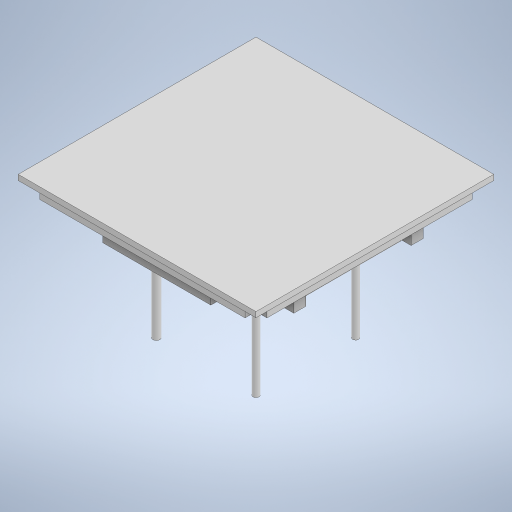
# Autodesk Inventor part: Acrilico_Bottom
Saved by Autodesk Inventor 2024 (Build 280153000, 153)
## iProperties
Created: 2023-06-25
Part Number: Acrilico_Bottom
Material: Genérico
Document SubType Name: Modeling
Designer: Personal
Density: 2.56911 g/cm^3
Appearance: Valor por defecto
Mass: 906.6 g
Surface Area: 1709.61 cm^2
Volume: 352.885 cm^3
Author: Personal
Autodesk Inventor part; units mm, degrees
ref_plane "YZ Plane" through (0, 0, 0) normal (1, 0, 0) x (0, 1, 0)
ref_plane "XZ Plane" through (0, 0, 0) normal (0, 1, 0) x (-1, 0, 0)
ref_plane "XY Plane" through (0, 0, 0) normal (0, 0, 1) x (1, 0, 0)
sketch "Boceto1" plane through (0, 0, 0) normal (0, 1, 0) x (-1, 0, 0)
  line L0 (-97.5, 97.5) -> (97.5, 97.5)
  line L1 (97.5, 97.5) -> (97.5, -97.5)
  line L2 (97.5, -97.5) -> (-97.5, -97.5)
  line L3 (-97.5, -97.5) -> (-97.5, 97.5)
  line L4 (-97.5, 97.5) -> (97.5, -97.5) construction
  line L5 (97.5, 97.5) -> (-97.5, -97.5) construction
  point P0 (0, 0)
  dimension "d0" = 195
  dimension "d1" = 195
  constraints: 12 end point, 2 midpoint, 2 parallel, 1 horizontal, 1 perpendicular
  measures "d0" distance of L0.end L1.end
  measures "d1" distance of L0.start L0.end
extrude "Extrusión1" add sketch "Boceto1" along normal mid plane 4.4
sketch "Boceto4" plane through (0, -2.2, 0) normal (0, -1, 0) x (1, 0, 0)
  line L0 (97.5, -97.5) -> (97.5, 97.5) construction
  line L1 (-97.5, 97.5) -> (-97.5, -97.5) construction
  line L2 (84.1, -93.1) -> (-84.1, -93.1)
  line L3 (-84.1, -93.1) -> (-84.1, -84.1)
  line L4 (-84.1, -84.1) -> (84.1, -84.1)
  line L5 (84.1, -84.1) -> (84.1, -93.1)
  line L6 (-97.5, -97.5) -> (97.5, -97.5) construction
  line L7 (93.1, -84.1) -> (84.1, -84.1)
  line L8 (84.1, -84.1) -> (84.1, 84.1)
  line L9 (84.1, 84.1) -> (93.1, 84.1)
  line L10 (93.1, 84.1) -> (93.1, -84.1)
  line L11 (0, -126.8945) -> (0, 107.949)
  line L12 (-84.1, -84.1) -> (-84.1, 84.1)
  line L13 (-84.1, 84.1) -> (-93.1, 84.1)
  line L14 (-93.1, 84.1) -> (-93.1, -84.1)
  line L15 (-93.1, -84.1) -> (-84.1, -84.1)
  line L16 (84.1, 84.1) -> (-84.1, 84.1)
  line L17 (84.1, 93.1) -> (-84.1, 93.1)
  line L18 (84.1, 84.1) -> (84.1, 93.1)
  line L19 (-84.1, 84.1) -> (-84.1, 93.1)
  point P0 (0, 0)
  point P1 (-84.1, -88.6)
  point P2 (88.6, -84.1)
  point P3 (84.1, -84.1)
  point P4 (84.1, -84.1)
  point P5 (84.1, -84.1)
  point P6 (84.1, -84.1)
  point P7 (-84.1, 84.1)
  point P8 (-84.1, 84.1)
  point P9 (-84.1, 84.1)
  point P10 (-84.1, 84.1)
  dimension "d20" = 4.4
  dimension "d21" = 9
  dimension "d22" = 13.4
  dimension "d23" = 13.4
  dimension "d24" = 4.4
  dimension "d25" = 9
  dimension "d26" = 13.4
  dimension "d30" = 9
  constraints: 34 end point, 5 horizontal, 4 parallel, 4 symmetric about line, 3 vertical, 2 midpoint, 2 perpendicular
  measures "d20" distance between parallel lines of L2 L6
  measures "d21" distance of L4.end L2.start
  measures "d22" distance between parallel lines of L0 L5
  measures "d23" distance from line of L1 point (-84.1, -88.6)
  measures "d24" distance between parallel lines of L0 L10
  measures "d25" distance of L7.start L7.end
  measures "d26" distance from line of point (88.6, -84.1) L6
  measures "d30" distance between parallel lines of L17 L16
extrude "Extrusión6" add sketch "Boceto4" along normal blind 9 contours L2 L11 L4 L5 | L2 L3 L4 L11 | L8 L9 L10 L7 | L16 L11 L17 L18 | L15 L14 L13 L12 | L16 L19 L17 L11
sketch "Boceto5" plane through (0, -11.2, 0) normal (0, -1, 0) x (1, 0, 0)
  line L0 (-84.1, -93.1) -> (84.1, -93.1) construction
  line L1 (93.1, -84.1) -> (93.1, 84.1) construction
  line L2 (-93.1, 84.1) -> (-93.1, -84.1) construction
  line L3 (84.1, 93.1) -> (-84.1, 93.1) construction
  line L4 (84.1, -93.1) -> (-84.1, -93.1)
  line L5 (-93.1, -84.1) -> (-93.1, 84.1)
  line L6 (-84.1, 93.1) -> (84.1, 93.1)
  line L7 (93.1, 84.1) -> (93.1, -84.1)
  line L8 (84.1, -93.1) -> (84.1, -84.1) projected
  line L9 (84.1, -84.1) -> (-84.1, -84.1) construction
  line L10 (84.1, -93.1) -> (84.1, -84.1)
  line L11 (84.1, -84.1) -> (93.1, -84.1)
  line L12 (93.1, 84.1) -> (84.1, 84.1)
  line L13 (84.1, 84.1) -> (84.1, 93.1)
  line L14 (-93.1, 84.1) -> (-84.1, 84.1)
  line L15 (-84.1, 84.1) -> (-84.1, 93.1)
  line L16 (-93.1, -84.1) -> (-84.1, -84.1) projected
  line L17 (-84.1, -93.1) -> (-84.1, -84.1)
  line L18 (-84.1, -84.1) -> (-93.1, -84.1)
  point P0 (0, 0)
  constraints: 24 end point, 9 point on line, 5 perpendicular, 2 horizontal, 2 parallel, 2 vertical
extrude "Extrusión7" add sketch "Boceto5" along normal blind 1.65
sketch "Boceto6" plane through (0, -12.85, 0) normal (0, -1, 0) x (1, 0, 0)
  line L0 (-84.1, -84.1) -> (84.1, -84.1) construction
  line L1 (53.1, -84.1) -> (43.1, -84.1)
  line L2 (43.1, -84.1) -> (43.1, -64.1)
  line L3 (43.1, -64.1) -> (53.1, -64.1)
  line L4 (53.1, -64.1) -> (53.1, -84.1)
  line L5 (93.1, -84.1) -> (93.1, 84.1) projected
  line L6 (84.1, -84.1) -> (84.1, 84.1) projected
  line L7 (64.1, -53.1) -> (84.1, -53.1)
  line L8 (84.1, -53.1) -> (84.1, -43.1)
  line L9 (84.1, -43.1) -> (64.1, -43.1)
  line L10 (64.1, -43.1) -> (64.1, -53.1)
  line L11 (-84.1, -93.1) -> (84.1, -93.1) projected
  point P0 (0, 0)
  dimension "d35" = 40
  dimension "d36" = 10
  dimension "d37" = 20
  dimension "d38" = 40
  dimension "d39" = 10
  dimension "d40" = 20
  constraints: 16 end point, 4 parallel, 2 horizontal, 2 perpendicular, 2 point on line
  measures "d35" distance between parallel lines of L5 L4
  measures "d36" distance of L2.end L3.end
  measures "d37" distance of L3.end L1.start
  measures "d38" distance between parallel lines of L11 L7
  measures "d39" distance of L9.end L7.start
  measures "d40" distance of L7.start L7.end
extrude "Extrusión8" add sketch "Boceto6" along normal blind 15
sketch "Boceto7" plane through (43.1, -12.85, -84.1) normal (-1, 0, 0) x (0, 0, 1)
  line L0 (0, 0) -> (20, 0) projected
  line L1 (0, 0) -> (0, -15) construction
  line L2 (20, -15) -> (0, -15) construction
  line L3 (20, 0) -> (20, -15) construction
  line L4 (0, 0) -> (20, 0) projected
  circle A0 centre (10, -7.5) radius 3.85
  point P0 (84.1, 12.85)
  dimension "d43" = 7.7
  constraints: 1 centre point
  measures "d43" diameter of A0
extrude "Extrusión9" add sketch "Boceto7" along normal blind 4
sketch "Boceto8" plane through (39.1, -20.35, -74.1) normal (-1, 0, 0) x (0, 0, 1)
  circle A0 centre (0, 0) radius 3.85 projected
  circle A1 centre (0, 0) radius 7.25
  point P0 (74.1, 20.35)
  dimension "d46" = 14.5
  constraints: 1 centre point, 1 coincident
  measures "d46" diameter of A1
extrude "Extrusión10" add sketch "Boceto8" along normal up to surface (39.1 mm away)
sketch "Boceto10" plane through (39.1, -20.35, -74.1) normal (-1, 0, 0) x (0, 0, 1)
  circle A0 centre (0, 0) radius 3.85 projected
  point P0 (74.1, 20.35)
extrude "Extrusión11" add sketch "Boceto10" along normal up to surface (39.1 mm away)
mirror "Simetría4" about plane through (0, 0, 0) normal (1, 0, 0) of "Extrusión9", "Extrusión10", "Extrusión11", "Extrusión8"
sketch "Boceto11" plane through (-84.1, -27.85, -53.1) normal (0, -1, 0) x (1, 0, 0)
  line L0 (20, 0) -> (0, 0) projected
  line L1 (20, 10) -> (20, 0) projected
  line L2 (0, 10) -> (20, 10) projected
  line L3 (0, 0) -> (0, 10) projected
  point P0 (84.1, 53.1)
extrude "Extrusión12" cut sketch "Boceto11" against normal up to surface (15 mm away)
sketch "Boceto12" plane through (64.1, -12.85, -43.1) normal (0, 0, 1) x (1, 0, 0)
  line L0 (0, 0) -> (20, 0) projected
  line L1 (0, 0) -> (0, -15) projected
  line L2 (20, -15) -> (0, -15) projected
  line L3 (20, 0) -> (20, -15) projected
  circle A0 centre (10, -7.5) radius 3.85
  point P0 (-64.1, 12.85)
  dimension "d53" = 7.7
  constraints: 1 centre point
  measures "d53" diameter of A0
extrude "Extrusión13" add sketch "Boceto12" along normal blind 4 contours A0
sketch "Boceto13" plane through (74.1, -20.35, -39.1) normal (0, 0, 1) x (1, 0, 0)
  circle A0 centre (0, 0) radius 3.85 projected
  circle A1 centre (0, 0) radius 7.25
  point P0 (-74.1, 20.35)
  dimension "d56" = 14.5
  constraints: 1 centre point, 1 coincident
  measures "d56" diameter of A1
extrude "Extrusión14" add sketch "Boceto13" along normal up to surface (39.1 mm away)
sketch "Boceto14" plane through (74.1, -20.35, -39.1) normal (0, 0, 1) x (1, 0, 0)
  circle A0 centre (0, 0) radius 3.85 projected
  point P0 (-74.1, 20.35)
extrude "Extrusión15" add sketch "Boceto14" along normal up to surface (39.1 mm away)
mirror "Simetría5" about plane through (0, 0, 0) normal (0, 0, 1) of "Extrusión15", "Extrusión14", "Extrusión13", "Extrusión12", "Extrusión8"
sketch "Boceto15" plane through (43.1, -27.85, 64.1) normal (0, -1, 0) x (1, 0, 0)
  line L0 (10, 0) -> (0, 0) projected
  line L1 (10, 20) -> (10, 0) projected
  line L2 (0, 20) -> (10, 20) projected
  line L3 (0, 0) -> (0, 20) projected
  point P0 (-43.1, -64.1)
extrude "Extrusión16" cut sketch "Boceto15" against normal up to surface (15 mm away)
sketch "Boceto16" plane through (0, -12.85, 0) normal (0, -1, 0) x (1, 0, 0)
  line L0 (81.35, 39.1) -> (66.85, 39.1) construction
  line L1 (81.35, -39.1) -> (66.85, -39.1) construction
  line L2 (81.35, -39.1) -> (81.35, 39.1) construction
  line L3 (66.85, -39.1) -> (66.85, 39.1) construction
  line L4 (81.35, -39.1) -> (66.85, -39.1) construction
  line L5 (81.35, 39.1) -> (66.85, 39.1) construction
  line L6 (-39.1, -66.85) -> (-39.1, -81.35) projected
  line L7 (39.1, -66.85) -> (39.1, -81.35) projected
  line L8 (-81.35, -44.335) -> (-66.85, -44.335)
  line L9 (-66.85, -44.335) -> (-66.85, 44.335)
  line L10 (-66.85, 44.335) -> (-81.35, 44.335)
  line L11 (-81.35, 44.335) -> (-81.35, -44.335)
  line L12 (-93.1, 84.1) -> (-93.1, -84.1) construction
  line L13 (84.1, 93.1) -> (-84.1, 93.1) construction
  line L14 (-44.335, 81.35) -> (-44.335, 66.85)
  line L15 (-44.335, 66.85) -> (44.335, 66.85)
  line L16 (44.335, 66.85) -> (44.335, 81.35)
  line L17 (44.335, 81.35) -> (-44.335, 81.35)
  point P0 (0, 0)
  dimension "d84" = 11.75
  dimension "d85" = 14.5
  dimension "d86" = 88.67
  dimension "d87" = 48.765
  dimension "d88" = 14.5
  dimension "d89" = 88.67
  dimension "d90" = 48.765
  dimension "d91" = 11.75
  constraints: 20 end point, 4 coincident, 4 parallel, 2 perpendicular, 1 horizontal
  measures "d84" distance between parallel lines of L11 L12
  measures "d85" distance of L8.start L8.end
  measures "d86" distance of L8.end L9.end
  measures "d87" distance between parallel lines of L13 L10
  measures "d88" distance of L14.start L15.start
  measures "d89" distance of L15.start L15.end
  measures "d90" distance between parallel lines of L12 L14
  measures "d91" distance between parallel lines of L13 L17
sketch "Boceto17" plane through (0, -12.85, 0) normal (0, -1, 0) x (1, 0, 0)
  line L0 (50.85, 50.85) -> (-50.85, 50.85) construction
  line L1 (-50.85, 50.85) -> (-50.85, -50.85) construction
  line L2 (-50.85, -50.85) -> (50.85, -50.85) construction
  line L3 (50.85, -50.85) -> (50.85, 50.85) construction
  line L4 (50.85, 50.85) -> (-50.85, -50.85) construction
  line L5 (-50.85, 50.85) -> (50.85, -50.85) construction
  circle A0 centre (40.85, 40.85) radius 2.5
  circle A1 centre (-40.85, 40.85) radius 2.8882
  line L6 (101.7, 0) -> (-109.1959, 0)
  circle A2 centre (40.85, -40.85) radius 2.5
  circle A3 centre (-40.85, -40.85) radius 2.8882
  point P0 (0, 0)
  dimension "d67" = 101.7
  dimension "d68" = 101.7
  dimension "d69" = 5
  dimension "d70" = 10
  dimension "d71" = 10
  dimension "d72" = 10
  dimension "d73" = 10
  constraints: 14 end point, 4 centre point, 2 horizontal, 2 midpoint, 2 parallel, 2 symmetric about line, 1 perpendicular, 2 other
  measures "d67" distance of L1.end L2.end
  measures "d68" distance of L2.end L0.start
  measures "d69" diameter of A0
  measures "d70" distance from line of L3 A0.centre
  measures "d71" distance from line of L0 A0.centre
  measures "d72" distance from line of L0 A1.centre
  measures "d73" distance from line of L1 A1.centre
extrude "Extrusión19" add sketch "Boceto17" along normal blind 100.95
sketch "Boceto18" plane through (0, -12.85, 0) normal (0, -1, 0) x (1, 0, 0)
  line L0 (84.1, 93.1) -> (-84.1, 93.1) projected
  line L1 (-84.1, 93.1) -> (-84.1, 84.1) projected
  line L2 (-84.1, 84.1) -> (-93.1, 84.1) projected
  line L3 (-93.1, 84.1) -> (-93.1, -84.1) projected
  line L4 (-93.1, -84.1) -> (-84.1, -84.1) projected
  line L5 (-84.1, -84.1) -> (-84.1, -93.1) projected
  line L6 (-84.1, -93.1) -> (84.1, -93.1) projected
  line L7 (84.1, -93.1) -> (84.1, -84.1) projected
  line L8 (93.1, -84.1) -> (93.1, 84.1) projected
  line L9 (84.1, -84.1) -> (93.1, -84.1) projected
  line L10 (93.1, 84.1) -> (84.1, 84.1) projected
  line L11 (84.1, 84.1) -> (84.1, 93.1) projected
  line L12 (-81.0533, 90.0533) -> (81.0533, 90.0533)
  line L13 (81.0533, 90.0533) -> (81.0533, 81.0533)
  line L14 (81.0533, 81.0533) -> (90.0533, 81.0533)
  line L15 (90.0533, 81.0533) -> (90.0533, -81.0533)
  line L16 (90.0533, -81.0533) -> (81.0533, -81.0533)
  line L17 (81.0533, -81.0533) -> (81.0533, -90.0533)
  line L18 (81.0533, -90.0533) -> (-81.0533, -90.0533)
  line L19 (-81.0533, -90.0533) -> (-81.0533, -81.0533)
  line L20 (-81.0533, -81.0533) -> (-90.0533, -81.0533)
  line L21 (-90.0533, -81.0533) -> (-90.0533, 81.0533)
  line L22 (-90.0533, 81.0533) -> (-81.0533, 81.0533)
  line L23 (-81.0533, 81.0533) -> (-81.0533, 90.0533)
  point P0 (0, 0)
  constraints: 24 end point, 11 other
extrude "Extrusión20" cut sketch "Boceto18" against normal blind 1.65
sketch "Boceto19" plane through (0, -12.85, 0) normal (0, -1, 0) x (1, 0, 0)
  circle A0 centre (-40.85, -40.85) radius 2.8882 construction
  circle A1 centre (-40.85, -40.85) radius 2.8882 construction
  circle A2 centre (-40.85, -40.85) radius 4
  line L0 (-66.85, -39.1) -> (-66.85, 39.1) projected
  circle A3 centre (-40.85, 40.85) radius 2.8882 construction
  circle A4 centre (-40.85, 40.85) radius 4
  line L1 (0, -105.6023) -> (0, 128.9456)
  circle A5 centre (40.85, -40.85) radius 2.8882 construction
  circle A6 centre (40.85, -40.85) radius 2.8882 construction
  circle A7 centre (40.85, -40.85) radius 4
  circle A8 centre (40.85, 40.85) radius 2.8882 construction
  circle A9 centre (40.85, 40.85) radius 4
  circle A10 centre (40.85, -40.85) radius 2.5 construction
  circle A11 centre (40.85, -40.85) radius 2.5 construction
  circle A12 centre (40.85, 40.85) radius 2.5 construction
  circle A13 centre (-40.85, 40.85) radius 2.8882 construction
  point P0 (0, 0)
  dimension "d78" = 8
  dimension "d79" = 8
  constraints: 7 centre point, 5 symmetric about line, 4 coincident, 3 concentric, 2 end point, 1 vertical, 5 other
  measures "d78" diameter of A2
  measures "d79" diameter of A4
extrude "Extrusión21" add sketch "Boceto19" along normal blind 19.1
extrude "Extrusión22" add sketch "Boceto16" along normal blind 15
